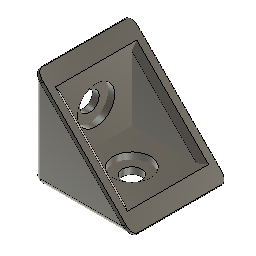
EXTRUSIONcorner (Autodesk Fusion 360 design; units mm, degrees)
part number: T-slot extrusion connectors
part number: CornerBracket
Autodesk Fusion 360 part; units mm, degrees
sketch "cornerSketch" plane through (0, 0, 0) normal (0, 1, 0) x (1, 0, 0) in component "body"
  line L0 (0, 0) -> (30, 0)
  line L1 (0, -30) -> (0, 0)
  line L2 (30, 0) -> (0, -30)
  dimension "d92" = 30
  dimension "d93" = 30
  constraint horizontal L0
  constraint vertical L1
  constraint coincident L0.start L1.end
  measures "d92" distance of L0.start L0.end
  measures "d93" distance of L0.start L1.start
extrude "Extrude6" add sketch "cornerSketch" along normal mid plane 30 in component "body"
shell "Shell1" thickness 4 removed faces 1 at (20, -5, 10) in component "body"
fillet "Fillet2" radius 2 5 edges at (0, 0, 0) (15, -15, 0) (0, -15, 15) (15, 15, 0) (0, 15, 15) in component "body"
chamfer "Chamfer4" distance 0.5 angle 45 8 edges at (0, 0, 30) (0.5858, 14.4142, 29.4142) (15, 15, 15) (29.4142, 14.4142, 0.5858) (30, 0, 0) (29.4142, -14.4142, 0.5858) (15, -15, 15) (0.5858, -14.4142, 29.4142) in component "body"
chamfer "Chamfer4" distance 1.5 angle 45 2 edges at (15, 11, 15) (15, -11, 15) in component "body"
sketch "oneSideSketch" plane through (0, 0, 4) normal (0, 0, 1) x (-1, 0, 0) in component "body"
  line L0 (-23.8787, -11) -> (-4, -11)
  line L1 (-4, -11) -> (-4, 11)
  line L2 (-4, 11) -> (-23.8787, 11)
  line L3 (-27, -4) -> (-3, -4)
  line L4 (-3, -4) -> (-3, 4)
  line L5 (-3, 4) -> (-27, 4)
  line L6 (-27, 4) -> (-27, -4)
  line L7 (-27, -4) -> (-3, 4) construction
  line L8 (-3, -4) -> (-27, 4) construction
  line L9 (-1.75, 0) -> (-22.5, 0)
  line L10 (-7, 4) -> (-23, 4)
  line L11 (-23, 4) -> (-23, -4)
  line L12 (-23, -4) -> (-7, -4)
  line L13 (-7, -4) -> (-7, 4)
  line L14 (-7, 4) -> (-23, -4) construction
  line L15 (-23, 4) -> (-7, -4) construction
  line L16 (-26, -12.5) -> (-23.8787, -11)
  line L17 (-23.8787, 11) -> (-26, 12.5)
  line L18 (-26, 12.5) -> (-26, -12.5)
  point P0 (-15, 0)
  point P1 (-15, 0)
  dimension "d134" = 24
  dimension "d135" = 8
  dimension "d136" = 15
  dimension "d137" = 16
  dimension "d138" = 8
  constraint horizontal L3
  constraint perpendicular L3 L4
  constraint parallel L3 L5
  constraint parallel L4 L6
  constraint coincident L7 P1
  constraint coincident L8 P1
  constraint coincident P1 L9
  constraint horizontal L10
  constraint perpendicular L10 L11
  constraint parallel L10 L12
  constraint parallel L11 L13
  constraint coincident L14 P1
  constraint coincident L15 P1
  constraint coincident P1 P0
  measures "d134" distance of L4.end L5.end
  measures "d135" distance of L3.end L4.end
  measures "d136" distance of origin P1
  measures "d137" distance of L11.end L12.end
  measures "d138" distance of L10.end L11.end
hole "Hole5" at (15, 0, 4) direction (0, 0, -1) diameter 6 depth 4 tip angle 180 counterbore diameter 11.5 counterbore depth 2 in component "body"
extrude "Extrude12" add sketch "oneSideSketch" against normal blind 2 from surface at -4 contours L1 L3 L9 L13 | L1 L3 L4 L9 | L3 L5 L11 L18 | L3 L5 L6 L18 | L1 L5 L9 L13 | L1 L4 L5 L9 in component "body"
chamfer "Chamfer6" distance 0.5 angle 45 2 faces at (4.3333, 1.3333, -2) (25.6667, 1.3333, -2) in component "body"
ref_plane "WorkPlane1" through (0, 12.125, 0) normal (0.707107, 0, -0.707107) x (0, 1, 0) in component "body"
mirror "Mirror2" about plane through (0, 12.125, 0) normal (0.707107, 0, -0.707107) of "Hole5", "Extrude12", "Chamfer6" in component "body"
pattern_linear "R-Pattern1" count 1 spacing 30 along (1, 0, 0) of "Hole5", "Extrude12", "Chamfer6" in component "body"
pattern_linear "R-Pattern2" count 1 spacing 30 along (0, 0, 1) of "Mirror2" in component "body"
component "body" placed x (1, 0, 0) y (0, 1, 0) z (0, 0, 1) at (0, 0, 0)
equation "size = 30 mm" comment "use 30 for 30x30 extrusions"
equation "d34 = size / 2"
equation "d92 = ( unitX * 30 ) * 1 mm"
equation "d93 = ( unitY * 30 ) * 1 mm"
equation "unitX = 1"
equation "unitY = 1"
equation "d145 = unitX"
equation "d147 = size"
equation "d150 = unitY"
equation "d152 = size"
named bodies: "bracket body"
